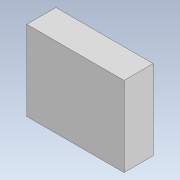
# Autodesk Inventor part: Блок питания LS-50-5_5V
Saved by Autodesk Inventor 2021.2 (Build 252289000, 289)
## iProperties
Created: 2022-11-29
Part Number: Блок питания LS-50-5_5V
Material: Типовые
Document SubType Name: Modeling
Designer: Voodoo
Mass: 246 g
Surface Area: 273.2 cm^2
Volume: 246 cm^3
Density: 1 g/cm^3
Appearance: По умолчанию
Author: Voodoo
Autodesk Inventor part; units mm, degrees
ref_plane "YZ Plane" through (0, 0, 0) normal (1, 0, 0) x (0, 1, 0)
ref_plane "XZ Plane" through (0, 0, 0) normal (0, 1, 0) x (-1, 0, 0)
ref_plane "XY Plane" through (0, 0, 0) normal (0, 0, 1) x (1, 0, 0)
sketch "Эскиз1" plane through (0, 0, 0) normal (0, 0, 1) x (1, 0, 0)
  line L0 (-50, -41) -> (50, -41)
  line L1 (50, -41) -> (50, 41)
  line L2 (50, 41) -> (-50, 41)
  line L3 (-50, 41) -> (-50, -41)
  line L4 (-50, -41) -> (50, 41) construction
  line L5 (50, -41) -> (-50, 41) construction
  point P0 (0, 0)
  dimension "d0" = 100
  dimension "d1" = 82
  constraints: 12 end point, 2 midpoint, 2 parallel, 1 horizontal, 1 perpendicular
  measures "d0" distance of L1.end L2.end
  measures "d1" distance of L2.end L0.start
extrude "Выдавливание1" add sketch "Эскиз1" along normal blind 30
